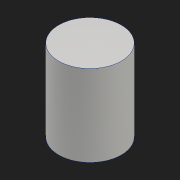
# Autodesk Inventor part: Odrive D5065
Saved by Autodesk Inventor 2017 (Build 210142000, 142)
## iProperties
Created: 2019-08-28
Part Number: Odrive D5065
Material: Aluminum 6061
Document SubType Name: Modeling
Designer: Dell
Density: 2.7 g/cm^3
Appearance: Aluminum - Flat
Mass: 344.593 g
Surface Area: 141.372 cm^2
Volume: 127.627 cm^3
Author: Dell
Autodesk Inventor part; units mm, degrees
ref_plane "YZ Plane" through (0, 0, 0) normal (1, 0, 0) x (0, 1, 0)
ref_plane "XZ Plane" through (0, 0, 0) normal (0, 1, 0) x (-1, 0, 0)
ref_plane "XY Plane" through (0, 0, 0) normal (0, 0, 1) x (1, 0, 0)
sketch "Sketch1" plane through (0, 0, 0) normal (0, 0, 1) x (1, 0, 0)
  circle A0 centre (0, 0) radius 25
  dimension "d0" = 50
  constraints: 1 centre point, 1 coincident
  measures "d0" diameter of A0
extrude "Extrusion1" add sketch "Sketch1" along normal blind 65
body "Solid1"
